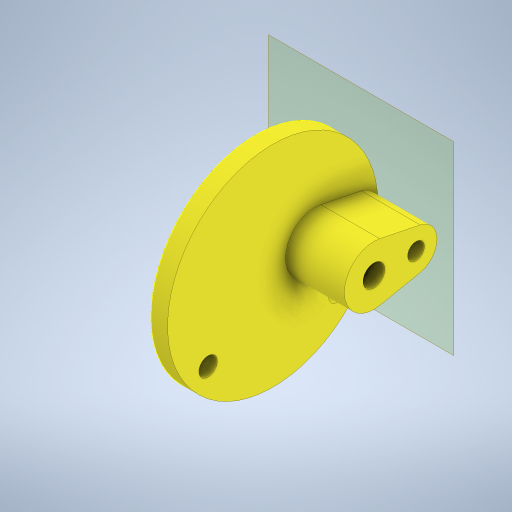
# Autodesk Inventor part: RSFF_mount_1_clearance
Saved by Autodesk Inventor 2023 (Build 270158000, 158)
## iProperties
Created: 2023-10-18
Part Number: RSFF_mount_1_clearance
Material: Generic
Document SubType Name: Modeling
Designer: MichihisaOohara
Density: 1 g/cm^3
Appearance: カナリア
Author: MichihisaOohara
Autodesk Inventor part; units mm, degrees
ref_plane "YZ Plane" through (0, 0, 0) normal (1, 0, 0) x (0, 1, 0)
ref_plane "XZ Plane" through (0, 0, 0) normal (0, 1, 0) x (-1, 0, 0)
ref_plane "XY Plane" through (0, 0, 0) normal (0, 0, 1) x (1, 0, 0)
sketch "スケッチ1" plane through (0, 0, 0) normal (1, 0, 0) x (0, 1, 0)
  circle A0 centre (0, 0) radius 10
  circle A1 centre (0, 0) radius 12.5
  circle A2 centre (0, -5) radius 1.3
  circle A3 centre (0, -10) radius 1
  circle A4 centre (0, -5) radius 3.5
  circle A5 centre (0, -10) radius 2.5
  circle A6 centre (-6.5, 7.7) radius 1.1
  circle A7 centre (-6.5, -7.7) radius 1.1
  line L0 (-6.5, 7.7) -> (-6.5, -7.7)
  line L1 (0, -5) -> (0, -10)
  line L2 (3.5006, -5.3506) -> (2.4495, -10.5)
  line L3 (-3.6097, -4.8161) -> (-2.4495, -10.5)
  dimension "d0" = 20
  dimension "d1" = 25
  dimension "d2" = 2.6
  dimension "d3" = 2
  dimension "d4" = 5
  dimension "d5" = 7
  dimension "d6" = 5
  dimension "d7" = 2.2
  dimension "d8" = 2.2
  dimension "d9" = 15.4
  dimension "d10" = 7.7
  dimension "d12" = 10
  dimension "d13" = 0
  dimension "d14" = 6.5
  dimension "d15" = 3.5
  dimension "d16" = 3.5
  constraints: 8 centre point, 8 end point, 4 coincident, 2 point on circle, 2 tangent, 2 vertical
  measures "d0" diameter of A0
  measures "d1" diameter of A1
  measures "d2" diameter of A2
  measures "d3" diameter of A3
  measures "d4" distance of A3.centre A2.centre
  measures "d5" diameter of A4
  measures "d6" diameter of A5
  measures "d7" diameter of A6
  measures "d8" diameter of A7
  measures "d9" distance of L0.start L0.end
  measures "d10" vertical distance of L0.start point (0, 0)
  measures "d12" distance of A1.centre A3.centre
  measures "d13" distance from line of L1 point (0, 0)
  measures "d14" distance from line of L0 point (0, 0)
  measures "d15" distance from line of L1.start L2
  measures "d16" distance from line of L1.start L3
extrude "押し出し1" add sketch "スケッチ1" against normal blind 2 contours A0 L2 A4 L3 A7 L0 A6 | A1 | L2 A5 A0 | A0 A5 A4 L2 | A6 L0 A7 A0 | A5 A0 A3 | A0 A3 L1 A4 A5 | A4 A5 | A4 L1 A5 | A3 A0 A5 A4 L1 | A4 A5 L1 | A4 A5 A0 L3 | L3 A0 A5
sketch "スケッチ2" plane through (0, 0, 0) normal (1, 0, 0) x (0, 0, -1)
  circle A0 centre (5, 0) radius 1.3 projected
  circle A1 centre (5, 0) radius 1.3
  circle A2 centre (5, 0) radius 3.5
  circle A3 centre (10, 0) radius 1 projected
  circle A4 centre (10, 0) radius 1
  circle A5 centre (10, 0) radius 2.5
  line L0 (10.9311, 2.3615) -> (5.7, 3.4293)
  line L1 (5.0718, -3.5575) -> (10.5, -2.4495)
  point P0 (0, 0)
  point P1 (5.7, -3.4293)
  point P2 (10.5, 2.4495)
  dimension "d19" = 7
  dimension "d20" = 5
  dimension "d21" = 2.5
  dimension "d22" = 3.5
  constraints: 4 coincident, 4 end point, 2 centre point, 8 other
  measures "d21" distance from line of point (10, 0) L0
  measures "d22" distance from line of point (5, 0) L1
extrude "押し出し2" add sketch "スケッチ2" along normal blind 7
sketch "スケッチ3" plane through (-2, 0, 0) normal (-1, 0, 0) x (0, 0, 1)
  circle A0 centre (-5, 0) radius 1.3 projected
  circle A1 centre (-5, 0) radius 1.3
  circle A2 centre (-5, 0) radius 2.4
  point P0 (0, 0)
  dimension "d25" = 4.8
  constraints: 2 centre point, 2 coincident
  measures "d25" diameter of A2
extrude "押し出し3" cut sketch "スケッチ3" against normal blind 5
sketch "スケッチ5" plane through (-2, 0, 0) normal (-1, 0, 0) x (0, 0, 1)
  circle A0 centre (0, 0) radius 12.5 projected
  point P0 (-12.5, 0)
  constraints: 1 horizontal alignment, 1 other
ref_plane "作業平面2" through (-2, 0, -12.5) normal (0, 0, -1) x (-1, 0, 0)
equation "\"d8\" = d7"
equation "\"d10\" = 0.5 * d9"
equation "\"d15\" = 0.5 * d5"
equation "\"d16\" = d15"
